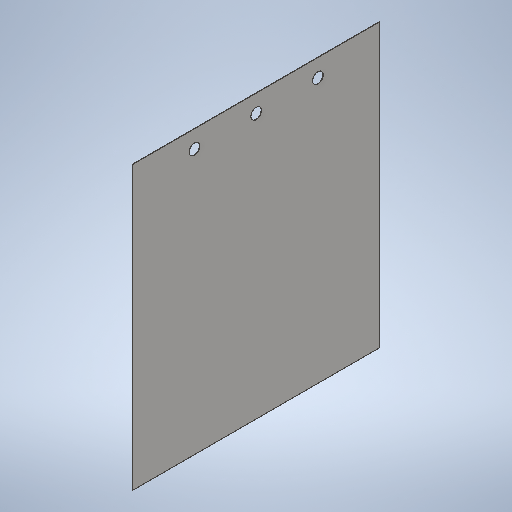
# Autodesk Inventor part: project Backrestfinal
Saved by Autodesk Inventor 2025.2 (Build 292293000, 293)
## iProperties
Created: 2025-02-04
Part Number: project Backrestfinal
Material: Steel, Galvanized
Document SubType Name: Sheet Metal
Designer: nandu
Density: 7.85 g/cm^3
Sheet Metal Rule: Default_mm
Appearance: Galvanized
Author: nandu
Autodesk Inventor part; units mm, degrees
ref_plane "YZ Plane" through (0, 0, 0) normal (1, 0, 0) x (0, 1, 0)
ref_plane "XZ Plane" through (0, 0, 0) normal (0, 1, 0) x (-1, 0, 0)
ref_plane "XY Plane" through (0, 0, 0) normal (0, 0, 1) x (1, 0, 0)
sketch "Sketch1" plane through (0, 0, 0) normal (1, 0, 0) x (0, 1, 0)
  line L0 (0, 0) -> (400, 0)
  line L1 (400, 0) -> (400, -350)
  line L2 (400, -350) -> (0, -350)
  line L3 (0, -350) -> (0, 0)
  dimension "d0" = 400
  dimension "d1" = 350
  constraints: 8 end point, 2 parallel, 1 horizontal, 1 perpendicular
  measures "d0" distance of L1.end L2.end
  measures "d1" distance of L0.end L1.end
extrude "Extrusion1" add sketch "Sketch1" along normal blind 0.607
sketch "Sketch2" plane through (0.607, 0, 0) normal (1, 0, 0) x (0, 0, -1)
  line L0 (0, 399.8291) -> (174.9999, 400)
  line L1 (350, 400) -> (0, 400) projected
  line L2 (174.9999, 400) -> (175.0243, 375)
  circle A0 centre (175.0243, 375) radius 7.5
  line L3 (175.0243, 375) -> (87.5243, 375)
  line L4 (175.0243, 375) -> (262.5243, 375)
  circle A1 centre (87.5243, 375) radius 7.5
  circle A2 centre (262.5243, 375) radius 7.5
  point P0 (0, 0)
  dimension "d4" = 175
  dimension "d5" = 25
  dimension "d7" = 15
  dimension "d12" = 15
  dimension "d13" = 15
  constraints: 8 end point, 3 centre point, 3 coincident, 2 horizontal, 1 midpoint, 1 perpendicular
  measures "d4" distance of L0.start L0.end
  measures "d5" distance of L0.end L2.end
  measures "d7" diameter of A0
  measures "d12" diameter of A1
  measures "d13" diameter of A2
extrude "Extrusion2" cut sketch "Sketch2" against normal through all
equation "\"BendRadius\" = Thickness"
equation "\"BendReliefWidth\" = Thickness"
equation "\"BendReliefDepth\" = 0.5 * Thickness"
equation "\"CornerReliefSize\" = 4 * Thickness"
equation "\"MinimumRemnant\" = 2 * Thickness"
equation "\"TransitionRadius\" = BendRadius"
equation "\"JacobiRadiusSize\" = BendRadius"
equation "\"GapSize\" = Thickness"
equation "\"Thickness\" = 0.607"
body "Solid1"
